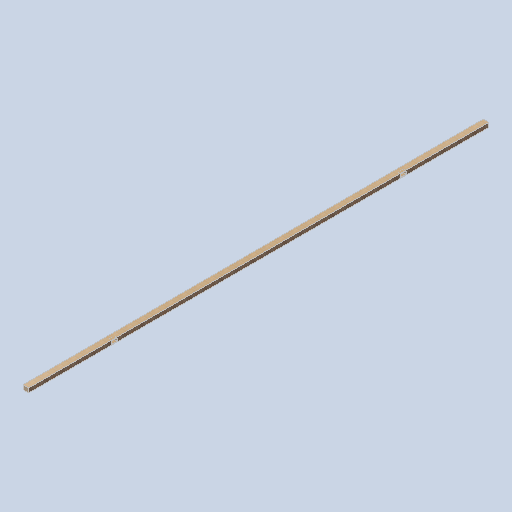
# Autodesk Inventor part: support_frame_01
Saved by Autodesk Inventor 2024.2 (Build 282272000, 272)
## iProperties
Created: 2024-05-22
Part Number: support_frame_01
Material: Wood (Maple)
Document SubType Name: Modeling
Designer: LOSTER_1
Density: 0.67 g/cm^3
Appearance: Natural Maple - Glossy Dark Tint
Author: LOSTER_1
Autodesk Inventor part; units mm, degrees
ref_plane "YZ Plane" through (0, 0, 0) normal (1, 0, 0) x (0, 1, 0)
ref_plane "XZ Plane" through (0, 0, 0) normal (0, 1, 0) x (-1, 0, 0)
ref_plane "XY Plane" through (0, 0, 0) normal (0, 0, 1) x (1, 0, 0)
sketch "Sketch1" plane through (0, 0, 0) normal (0, 0, 1) x (1, 0, 0)
  line L0 (-817.1803, 145.656) -> (-1217.1803, 145.656)
  line L1 (-1217.1803, 145.656) -> (-1217.1803, -156.5826)
  line L2 (-1217.1803, -156.5826) -> (-817.1803, -156.5826)
  line L3 (-817.1803, -156.5826) -> (-817.1803, 145.656)
  point P0 (0, 0)
  point P1 (-1217.1803, -156.5826)
  point P2 (782.8197, 145.656)
  point P3 (1182.8197, -156.5826)
  constraints: 8 end point, 2 coincident, 2 parallel, 1 horizontal, 1 perpendicular
extrude "Extrusion1" add sketch "Sketch1" along normal blind 32302
sketch "Sketch2" plane through (-817.1803, 145.656, 32302) normal (1, 0, 0) x (0, 0, -1)
  line L0 (6000, 0) -> (6000, -302.2386)
  line L1 (5800, -51.1193) -> (6200, -51.1193)
  line L2 (6200, -51.1193) -> (6200, -251.1193)
  line L3 (6200, -251.1193) -> (5800, -251.1193)
  line L4 (5800, -251.1193) -> (5800, -51.1193)
  line L5 (5800, -51.1193) -> (6200, -251.1193) construction
  line L6 (6200, -51.1193) -> (5800, -251.1193) construction
  line L7 (16151, 0) -> (16151, -447.3568)
  line L8 (26302, 0) -> (26302, -302.2386)
  line L9 (26502, -51.1193) -> (26102, -51.1193)
  line L10 (26102, -51.1193) -> (26102, -251.1193)
  line L11 (26102, -251.1193) -> (26502, -251.1193)
  line L12 (26502, -251.1193) -> (26502, -51.1193)
  line L13 (26502, -51.1193) -> (26102, -251.1193) construction
  line L14 (26102, -51.1193) -> (26502, -251.1193) construction
  point P0 (32302, -145.656)
  point P1 (0, 0)
  point P2 (6000, -151.1193)
  point P3 (26302, -151.1193)
  dimension "d3" = 400
  dimension "d4" = 200
  constraints: 30 end point, 8 symmetric about line, 3 midpoint, 2 coincident, 2 parallel, 1 horizontal, 1 perpendicular, 1 vertical
  measures "d3" distance of L2.end L3.end
  measures "d4" distance of L1.end L2.end
extrude "Extrusion2" cut sketch "Sketch2" against normal blind 200
body "Solid1"
